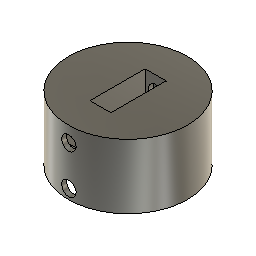
base_bottom (Autodesk Fusion 360 design; units mm, degrees)
Autodesk Fusion 360 part; units mm, degrees
sketch "Sketch1" plane through (0, 0, 0) normal (0, 0, 1) x (1, 0, 0)
  line L0 (34.925, 31.75) -> (-34.925, 31.75)
  line L1 (-34.925, 31.75) -> (-34.925, -31.75)
  line L2 (-34.925, -31.75) -> (34.925, -31.75)
  line L3 (34.925, -31.75) -> (34.925, 31.75)
  line L4 (34.925, 31.75) -> (-34.925, -31.75) construction
  line L5 (-34.925, 31.75) -> (34.925, -31.75) construction
  circle A0 centre (0, 0) radius 62.5
  dimension "d1" = 69.85
  dimension "d2" = 63.5
  dimension "d3" = 125
  constraint horizontal L0
  constraint perpendicular L0 L1
  constraint parallel L0 L2
  constraint parallel L1 L3
  constraint coincident L4 A0.centre
  constraint coincident L5 A0.centre
  constraint coincident A0.centre origin
  measures "d1" distance of L1.end L2.end
  measures "d2" distance of L0.end L1.end
  measures "d3" diameter of A0
extrude "Extrude1" add sketch "Sketch1" along normal blind 31.75 contours L0 L1 L2 L3 | A0 makes body 1
extrude "Extrude2" cut sketch "Sketch1" along normal blind 20.32 contours L0 L1 L2 L3 bodies 1
sketch "Sketch3" plane through (0, 0, 31.75) normal (0, 0, 1) x (-1, 0, 0)
  circle A0 centre (0, 0) radius 62.5
  line L0 (-11, 29) -> (11, 29)
  line L1 (11, 29) -> (11, -29)
  line L2 (11, -29) -> (-11, -29)
  line L3 (-11, -29) -> (-11, 29)
  line L4 (-11, 29) -> (11, -29) construction
  line L5 (11, 29) -> (-11, -29) construction
  circle A1 centre (0, 0) radius 35
  dimension "d23" = 22
  dimension "d24" = 58
  dimension "d25" = 70
  constraint horizontal L0
  constraint perpendicular L0 L1
  constraint parallel L0 L2
  constraint parallel L1 L3
  constraint coincident L4 A0.centre
  constraint coincident L5 A0.centre
  constraint coincident A0.centre A1.centre
  measures "d23" distance of L1.end L2.end
  measures "d24" distance of L0.end L1.end
  measures "d25" diameter of A1
extrude "Extrude4" add sketch "Sketch3" along normal blind 36 contours A1 bodies 1
extrude "Extrude5" add 1 faces at (52.9703, -4.8439, 31.75) along direction (0, 0, 1) blind 36 on bodies 1 bodies 1
shell "Shell2" thickness 5 removed faces 1 at (-1.5569, -41.9417, 0) on bodies 1 makes body 2 at (-5.3333, 11.3333, 25.32)
sketch "Sketch4" plane through (0, 29, 0) normal (0, -1, 0) x (1, 0, 0)
  line L0 (-11, 31.75) -> (11, 31.75)
  line L1 (11, 31.75) -> (11, 67.75)
  line L2 (11, 67.75) -> (-11, 67.75)
  line L3 (-11, 67.75) -> (-11, 31.75)
  line L4 (0, 31.75) -> (0, 67.75)
  circle A0 centre (0, 51.5885) radius 7.5
  dimension "d31" = 15
  constraint midpoint L0 L4.start
  constraint midpoint L2 L4.end
  constraint coincident L4 A0.centre
  measures "d31" diameter of A0
extrude "Extrude6" cut sketch "Sketch4" along normal mid plane 200 contours L4 A0 | L4 A0 bodies 1
sketch "Sketch5" plane through (0, 31.75, 0) normal (0, -1, 0) x (1, 0, 0)
  line L0 (-34.925, 0) -> (34.925, 0)
  line L1 (34.925, 0) -> (34.925, 20.32)
  line L2 (34.925, 20.32) -> (-34.925, 20.32)
  line L3 (-34.925, 20.32) -> (-34.925, 0)
  line L4 (-34.925, 20.32) -> (34.925, 20.32)
  line L5 (34.925, 20.32) -> (34.925, 0)
  line L6 (34.925, 0) -> (-34.925, 0)
  line L7 (-34.925, 0) -> (-34.925, 20.32)
  line L8 (-34.925, 20.32) -> (34.925, 0) construction
  line L9 (34.925, 20.32) -> (-34.925, 0) construction
  circle A0 centre (0, 10.16) radius 7.5
  dimension "d34" = 15
  constraint horizontal L4
  constraint vertical L5
  constraint horizontal L6
  constraint vertical L7
  constraint coincident L0.end L1.start
  constraint coincident L2.end L3.start
  constraint coincident L1.end L2.start
  constraint coincident L0.start L3.end
  constraint midpoint L9 A0.centre
  measures "d34" diameter of A0
extrude "Extrude7" cut sketch "Sketch5" along normal mid plane 400 contours A0 bodies 1 2
